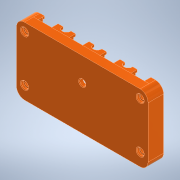
# Autodesk Inventor part: casing-top
Saved by Autodesk Inventor 2021 (Build 250183000, 183)
## iProperties
Created: 2022-04-08
Part Number: casing-top
Material: PET Plastic
Document SubType Name: Modeling
Designer: Staňa
Density: 1.541 g/cm^3
Appearance: Smooth - Light Orange
Author: Staňa
Autodesk Inventor part; units mm, degrees
ref_plane "YZ Plane" through (0, 0, 0) normal (1, 0, 0) x (0, 1, 0)
ref_plane "XZ Plane" through (0, 0, 0) normal (0, 1, 0) x (-1, 0, 0)
ref_plane "XY Plane" through (0, 0, 0) normal (0, 0, 1) x (1, 0, 0)
sketch "Sketch1" plane through (0, 0, 0) normal (0, 0, 1) x (1, 0, 0)
  line L0 (-46.7497, 20.955) -> (-42.9801, 20.955) construction
  line L1 (-42.9801, 20.955) -> (-42.9801, 22.455) construction
  line L2 (-42.9801, 22.455) -> (-46.7497, 22.455) projected
  arc A0 (-46.7497, 22.455) -> (-51.75, 17.4547) centre (-46.7497, 17.4547) ccw projected
  line L3 (-51.75, 17.4547) -> (-51.75, -19.9997) projected
  arc A1 (-51.75, -19.9997) -> (-46.7497, -25) centre (-46.7497, -19.9997) ccw projected
  line L4 (-46.7497, -25) -> (-35.7299, -25) projected
  line L5 (-35.7299, -25) -> (-35.7299, -23.5) construction
  line L6 (-35.7299, -23.5) -> (-46.7497, -23.5) construction
  arc A2 (-50.25, -19.9997) -> (-46.7497, -23.5) centre (-46.7497, -19.9997) ccw construction
  line L7 (-50.25, -19.9997) -> (-50.25, 17.4547) construction
  arc A3 (-46.7497, 20.955) -> (-50.25, 17.4547) centre (-46.7497, 17.4547) ccw construction
  line L8 (-27.98, 20.955) -> (-27.98, 22.455) construction
  line L9 (-27.98, 22.455) -> (-32.0201, 22.455) projected
  line L10 (-32.0201, 22.455) -> (-32.0201, 20.955) construction
  line L11 (-32.0201, 20.955) -> (-27.98, 20.955) construction
  line L12 (-21.63, 22.455) -> (-21.63, 20.955) construction
  line L13 (-21.63, 20.955) -> (-17.9801, 20.955) construction
  line L14 (-17.9801, 20.955) -> (-17.9801, 22.455) construction
  line L15 (-17.9801, 22.455) -> (-21.63, 22.455) projected
  line L16 (-2.98, 20.955) -> (-2.98, 22.455) construction
  line L17 (-2.98, 22.455) -> (-7.0201, 22.455) projected
  line L18 (-7.0201, 22.455) -> (-7.0201, 20.955) construction
  line L19 (-7.0201, 20.955) -> (-2.98, 20.955) construction
  line L20 (3.37, 22.455) -> (3.37, 20.955) construction
  line L21 (3.37, 20.955) -> (7.0199, 20.955) construction
  line L22 (7.0199, 20.955) -> (7.0199, 22.455) construction
  line L23 (7.0199, 22.455) -> (3.37, 22.455) projected
  line L24 (22.02, 20.955) -> (22.02, 22.455) construction
  line L25 (22.02, 22.455) -> (17.9799, 22.455) projected
  line L26 (17.9799, 22.455) -> (17.9799, 20.955) construction
  line L27 (17.9799, 20.955) -> (22.02, 20.955) construction
  line L28 (28.37, 22.455) -> (28.37, 20.955) construction
  line L29 (28.37, 20.955) -> (32.0199, 20.955) construction
  line L30 (32.0199, 20.955) -> (32.0199, 22.455) construction
  line L31 (32.0199, 22.455) -> (28.37, 22.455) projected
  line L32 (50.25, 17.4547) -> (50.25, -19.9997) construction
  arc A4 (46.7497, -23.5) -> (50.25, -19.9997) centre (46.7497, -19.9997) ccw construction
  line L33 (46.7497, -23.5) -> (35.7301, -23.5) construction
  line L34 (35.7301, -23.5) -> (35.7301, -25) construction
  line L35 (35.7301, -25) -> (46.7497, -25) projected
  arc A5 (46.7497, -25) -> (51.75, -19.9997) centre (46.7497, -19.9997) ccw projected
  line L36 (51.75, -19.9997) -> (51.75, 17.4547) projected
  arc A6 (51.75, 17.4547) -> (46.7497, 22.455) centre (46.7497, 17.4547) ccw projected
  line L37 (46.7497, 22.455) -> (42.9799, 22.455) projected
  line L38 (42.9799, 22.455) -> (42.9799, 20.955) construction
  line L39 (42.9799, 20.955) -> (46.7497, 20.955) construction
  arc A7 (50.25, 17.4547) -> (46.7497, 20.955) centre (46.7497, 17.4547) ccw construction
  arc A8 (-46.7497, 24.2499) -> (-53.25, 17.7496) centre (-46.7497, 17.7496) ccw projected
  line L40 (-53.25, 17.7496) -> (-53.25, -23.7996) projected
  arc A9 (-53.25, -23.7996) -> (-46.7497, -30.2999) centre (-46.7497, -23.7996) ccw projected
  line L41 (-46.7497, -30.2999) -> (46.7497, -30.2999) projected
  arc A10 (46.7497, -30.2999) -> (53.25, -23.7996) centre (46.7497, -23.7996) ccw projected
  line L42 (53.25, -23.7996) -> (53.25, 17.7496) projected
  arc A11 (53.25, 17.7496) -> (46.7497, 24.2499) centre (46.7497, 17.7496) ccw projected
  line L43 (46.7497, 24.2499) -> (42.9799, 24.2499)
  line L44 (42.9799, 24.2499) -> (42.9799, 22.455)
  line L45 (-46.7497, 24.2499) -> (-42.9801, 24.2499)
  line L46 (-42.9801, 24.2499) -> (-42.9801, 22.455)
  line L47 (-35.7299, -25) -> (-35.7299, -30.2999)
  line L48 (35.7301, -25) -> (35.7301, -30.2999)
  line L49 (-32.0201, 22.455) -> (-17.9801, 22.455)
  line L50 (-17.9801, 22.455) -> (-17.9801, 24.2499)
  line L51 (-17.9801, 24.2499) -> (-32.0201, 24.2499)
  line L52 (-32.0201, 24.2499) -> (-32.0201, 22.455)
  line L53 (-7.0201, 22.455) -> (7.0199, 22.455)
  line L54 (7.0199, 22.455) -> (7.0199, 24.2499)
  line L55 (7.0199, 24.2499) -> (-7.0201, 24.2499)
  line L56 (-7.0201, 24.2499) -> (-7.0201, 22.455)
  line L57 (17.9799, 22.455) -> (32.0199, 22.455)
  line L58 (32.0199, 22.455) -> (32.0199, 24.2499)
  line L59 (32.0199, 24.2499) -> (17.9799, 24.2499)
  line L60 (17.9799, 24.2499) -> (17.9799, 22.455)
  constraints: 36 end point, 7 perpendicular, 6 parallel, 5 horizontal, 5 point on line, 3 collinear
extrude "bottom-indent" add sketch "Sketch1" along normal blind 1.5
sketch "Sketch3" plane through (0, 0, 1.5) normal (0, 0, 1) x (1, 0, 0)
  arc A0 (-51.75, -19.9997) -> (-46.7497, -25) centre (-46.7497, -19.9997) ccw
  line L0 (-51.75, -19.9997) -> (-51.75, 17.4547)
  arc A1 (-46.7497, 22.455) -> (-51.75, 17.4547) centre (-46.7497, 17.4547) ccw
  line L1 (-46.7497, 22.455) -> (-42.9801, 22.455) construction
  line L2 (-42.9801, 22.455) -> (-42.9801, 24.2499)
  line L3 (-42.9801, 24.2499) -> (-46.7497, 24.2499)
  arc A2 (-46.7497, 24.2499) -> (-53.25, 17.7496) centre (-46.7497, 17.7496) ccw
  line L4 (-53.25, 17.7496) -> (-53.25, -23.7996)
  arc A3 (-53.25, -23.7996) -> (-46.7497, -30.2999) centre (-46.7497, -23.7996) ccw
  line L5 (-46.7497, -30.2999) -> (-35.7299, -30.2999)
  line L6 (-35.7299, -30.2999) -> (-35.7299, -25)
  line L7 (-35.7299, -25) -> (-46.7497, -25)
  line L8 (-46.7497, 20.955) -> (-42.9801, 20.955)
  line L9 (-42.9801, 20.955) -> (-42.9801, 22.455)
  line L10 (-42.9801, 22.455) -> (-46.7497, 22.455) construction
  arc A4 (-46.7497, 22.455) -> (-51.75, 17.4547) centre (-46.7497, 17.4547) ccw
  line L11 (-51.75, 17.4547) -> (-51.75, -19.9997)
  arc A5 (-51.75, -19.9997) -> (-46.7497, -25) centre (-46.7497, -19.9997) ccw
  line L12 (-46.7497, -25) -> (-35.7299, -25)
  line L13 (-35.7299, -25) -> (-35.7299, -23.5)
  line L14 (-35.7299, -23.5) -> (-46.7497, -23.5)
  arc A6 (-50.25, -19.9997) -> (-46.7497, -23.5) centre (-46.7497, -19.9997) ccw
  line L15 (-50.25, -19.9997) -> (-50.25, 17.4547)
  arc A7 (-46.7497, 20.955) -> (-50.25, 17.4547) centre (-46.7497, 17.4547) ccw
  line L16 (-32.0201, 22.455) -> (-17.9801, 22.455) construction
  line L17 (-17.9801, 22.455) -> (-17.9801, 24.2499)
  line L18 (-17.9801, 24.2499) -> (-32.0201, 24.2499)
  line L19 (-32.0201, 24.2499) -> (-32.0201, 22.455)
  line L20 (-7.0201, 22.455) -> (7.0199, 22.455) construction
  line L21 (7.0199, 22.455) -> (7.0199, 24.2499)
  line L22 (7.0199, 24.2499) -> (-7.0201, 24.2499)
  line L23 (-7.0201, 24.2499) -> (-7.0201, 22.455)
  line L24 (17.9799, 22.455) -> (32.0199, 22.455) construction
  line L25 (32.0199, 22.455) -> (32.0199, 24.2499)
  line L26 (32.0199, 24.2499) -> (17.9799, 24.2499)
  line L27 (17.9799, 24.2499) -> (17.9799, 22.455)
  line L28 (35.7301, -25) -> (35.7301, -30.2999)
  line L29 (35.7301, -30.2999) -> (46.7497, -30.2999)
  arc A8 (46.7497, -30.2999) -> (53.25, -23.7996) centre (46.7497, -23.7996) ccw
  line L30 (53.25, -23.7996) -> (53.25, 17.7496)
  arc A9 (53.25, 17.7496) -> (46.7497, 24.2499) centre (46.7497, 17.7496) ccw
  line L31 (46.7497, 24.2499) -> (42.9799, 24.2499)
  line L32 (42.9799, 24.2499) -> (42.9799, 22.455)
  line L33 (42.9799, 22.455) -> (46.7497, 22.455) construction
  arc A10 (51.75, 17.4547) -> (46.7497, 22.455) centre (46.7497, 17.4547) ccw
  line L34 (51.75, 17.4547) -> (51.75, -19.9997)
  arc A11 (46.7497, -25) -> (51.75, -19.9997) centre (46.7497, -19.9997) ccw
  line L35 (46.7497, -25) -> (35.7301, -25)
  line L36 (50.25, 17.4547) -> (50.25, -19.9997)
  arc A12 (46.7497, -23.5) -> (50.25, -19.9997) centre (46.7497, -19.9997) ccw
  line L37 (46.7497, -23.5) -> (35.7301, -23.5)
  line L38 (35.7301, -23.5) -> (35.7301, -25)
  line L39 (35.7301, -25) -> (46.7497, -25)
  arc A13 (46.7497, -25) -> (51.75, -19.9997) centre (46.7497, -19.9997) ccw
  line L40 (51.75, -19.9997) -> (51.75, 17.4547)
  arc A14 (51.75, 17.4547) -> (46.7497, 22.455) centre (46.7497, 17.4547) ccw
  line L41 (46.7497, 22.455) -> (42.9799, 22.455) construction
  line L42 (42.9799, 22.455) -> (42.9799, 20.955)
  line L43 (42.9799, 20.955) -> (46.7497, 20.955)
  arc A15 (50.25, 17.4547) -> (46.7497, 20.955) centre (46.7497, 17.4547) ccw
  line L44 (-32.0201, 24.2499) -> (-32.0201, 22.455)
  line L45 (-32.0201, 24.2499) -> (-17.9801, 24.2499)
  line L46 (-17.9801, 24.2499) -> (-17.9801, 20.955)
  line L47 (-17.9801, 20.955) -> (-32.0201, 20.955)
  line L48 (-32.0201, 20.955) -> (-32.0201, 24.2499)
  line L49 (-17.9801, 22.455) -> (-17.9801, 24.2499)
  line L50 (7.0199, 24.2499) -> (-7.0201, 24.2499)
  line L51 (-7.0201, 24.2499) -> (7.0199, 24.2499)
  line L52 (7.0199, 24.2499) -> (7.0199, 20.955)
  line L53 (7.0199, 20.955) -> (-7.0201, 20.955)
  line L54 (-7.0201, 20.955) -> (-7.0201, 24.2499)
  line L55 (32.0199, 24.2499) -> (17.9799, 24.2499)
  line L56 (17.9799, 24.2499) -> (32.0199, 24.2499)
  line L57 (32.0199, 24.2499) -> (32.0199, 20.955)
  line L58 (32.0199, 20.955) -> (17.9799, 20.955)
  line L59 (17.9799, 20.955) -> (17.9799, 24.2499)
  line L60 (32.0199, 22.455) -> (32.0199, 24.2499)
  line L61 (7.0199, 22.455) -> (7.0199, 24.2499)
  point P0 (0, 0)
extrude "dut-conn-wall" add sketch "Sketch3" along normal blind 3.7
sketch "Sketch4" plane through (0, 0, 5.2) normal (0, 0, 1) x (1, 0, 0)
  line L0 (-35.7299, -23.5) -> (-46.7497, -23.5) projected
  arc A0 (-50.25, -19.9997) -> (-46.7497, -23.5) centre (-46.7497, -19.9997) ccw projected
  line L1 (-50.25, -19.9997) -> (-50.25, 17.4547) projected
  arc A1 (-46.7497, 20.955) -> (-50.25, 17.4547) centre (-46.7497, 17.4547) ccw projected
  line L2 (-46.7497, 20.955) -> (-42.9801, 20.955) projected
  line L3 (-42.9801, 20.955) -> (-42.9801, 24.2499) construction
  line L4 (-42.9801, 24.2499) -> (-46.7497, 24.2499) projected
  arc A2 (-46.7497, 24.2499) -> (-53.25, 17.7496) centre (-46.7497, 17.7496) ccw projected
  line L5 (-53.25, 17.7496) -> (-53.25, -23.7996) projected
  arc A3 (-53.25, -23.7996) -> (-46.7497, -30.2999) centre (-46.7497, -23.7996) ccw projected
  line L6 (-46.7497, -30.2999) -> (-35.7299, -30.2999) projected
  line L7 (-35.7299, -30.2999) -> (-35.7299, -23.5) projected
  line L8 (35.7301, -30.2999) -> (46.7497, -30.2999) projected
  arc A4 (46.7497, -30.2999) -> (53.25, -23.7996) centre (46.7497, -23.7996) ccw projected
  line L9 (53.25, -23.7996) -> (53.25, 17.7496) projected
  arc A5 (53.25, 17.7496) -> (46.7497, 24.2499) centre (46.7497, 17.7496) ccw projected
  line L10 (46.7497, 24.2499) -> (42.9799, 24.2499) projected
  line L11 (42.9799, 24.2499) -> (42.9799, 20.955) construction
  line L12 (42.9799, 20.955) -> (46.7497, 20.955) projected
  arc A6 (50.25, 17.4547) -> (46.7497, 20.955) centre (46.7497, 17.4547) ccw projected
  line L13 (50.25, 17.4547) -> (50.25, -19.9997) projected
  arc A7 (46.7497, -23.5) -> (50.25, -19.9997) centre (46.7497, -19.9997) ccw projected
  line L14 (46.7497, -23.5) -> (35.7301, -23.5) projected
  line L15 (35.7301, -23.5) -> (35.7301, -30.2999) projected
  line L16 (-42.9801, 24.2499) -> (-46.7497, 24.2499) projected
  line L17 (46.7497, 24.2499) -> (42.9799, 24.2499) projected
  line L18 (-42.9801, 24.2499) -> (42.9799, 24.2499)
  line L19 (42.9799, 20.955) -> (-42.9801, 20.955)
  point P0 (0, 0)
  constraints: 4 end point, 1 collinear, 1 horizontal
extrude "mso-conn-wall" add sketch "Sketch4" along normal blind 4.15
sketch "Sketch5" plane through (0, 0, 9.35) normal (0, 0, 1) x (1, 0, 0)
  line L0 (46.7497, 24.2499) -> (-46.7497, 24.2499) projected
  arc A0 (-46.7497, 24.2499) -> (-53.25, 17.7496) centre (-46.7497, 17.7496) ccw projected
  line L1 (-53.25, 17.7496) -> (-53.25, -23.7996) projected
  arc A1 (-53.25, -23.7996) -> (-46.7497, -30.2999) centre (-46.7497, -23.7996) ccw projected
  line L2 (-46.7497, -30.2999) -> (-35.7299, -30.2999) projected
  line L3 (-35.7299, -30.2999) -> (-35.7299, -23.5) construction
  line L4 (-35.7299, -23.5) -> (-46.7497, -23.5) projected
  arc A2 (-50.25, -19.9997) -> (-46.7497, -23.5) centre (-46.7497, -19.9997) ccw projected
  line L5 (-50.25, -19.9997) -> (-50.25, 17.4547) projected
  arc A3 (-46.7497, 20.955) -> (-50.25, 17.4547) centre (-46.7497, 17.4547) ccw projected
  line L6 (-46.7497, 20.955) -> (46.7497, 20.955) projected
  arc A4 (50.25, 17.4547) -> (46.7497, 20.955) centre (46.7497, 17.4547) ccw projected
  line L7 (50.25, 17.4547) -> (50.25, -19.9997) projected
  arc A5 (46.7497, -23.5) -> (50.25, -19.9997) centre (46.7497, -19.9997) ccw projected
  line L8 (46.7497, -23.5) -> (35.7301, -23.5) projected
  line L9 (35.7301, -23.5) -> (35.7301, -30.2999) construction
  line L10 (35.7301, -30.2999) -> (46.7497, -30.2999) projected
  arc A6 (46.7497, -30.2999) -> (53.25, -23.7996) centre (46.7497, -23.7996) ccw projected
  line L11 (53.25, -23.7996) -> (53.25, 17.7496) projected
  arc A7 (53.25, 17.7496) -> (46.7497, 24.2499) centre (46.7497, 17.7496) ccw projected
  line L12 (-46.7497, -30.2999) -> (-35.7299, -30.2999) projected
  line L13 (-35.7299, -30.2999) -> (35.7301, -30.2999)
  line L14 (-35.7299, -23.5) -> (-46.7497, -23.5) construction
  line L15 (-35.7299, -30.2999) -> (-35.7299, -23.5) construction
  line L16 (-35.7299, -23.5) -> (-46.7497, -23.5) projected
  line L17 (46.7497, -23.5) -> (35.7301, -23.5) projected
  point P0 (0, 0)
  constraints: 2 end point, 1 horizontal
extrude "roof" add sketch "Sketch5" along normal blind 3.15
sketch "Sketch7" plane through (-7.0201, 24.2499, 0) normal (0, 1, 0) x (1, 0, 0)
  circle A0 centre (32.0201, -0.255) radius 3.25 construction
  arc A1 (29.2901, -1.7655) -> (29.2901, 1.2555) centre (32.0201, -0.255) ccw construction
  line L0 (29.2901, -1.7655) -> (29.2901, 1.2555) construction
  circle A2 centre (7.0201, -0.255) radius 3.25 construction
  arc A3 (4.2901, -1.7655) -> (4.2901, 1.2555) centre (7.0201, -0.255) ccw construction
  line L1 (4.2901, -1.7655) -> (4.2901, 1.2555) construction
  circle A4 centre (-17.9799, -0.255) radius 3.25 construction
  arc A5 (-20.7099, -1.7655) -> (-20.7099, 1.2555) centre (-17.9799, -0.255) ccw construction
  line L2 (-20.7099, -1.7655) -> (-20.7099, 1.2555) construction
  arc A6 (29.0401, -1.8287) -> (29.0401, 1.3187) centre (32.0201, -0.255) ccw
  line L3 (29.0401, -1.8287) -> (29.0401, 1.3187)
  arc A7 (4.0401, -1.8287) -> (4.0401, 1.3187) centre (7.0201, -0.255) ccw
  line L4 (4.0401, -1.8287) -> (4.0401, 1.3187)
  arc A8 (-20.9599, -1.8287) -> (-20.9599, 1.3187) centre (-17.9799, -0.255) ccw
  line L5 (-20.9599, -1.8287) -> (-20.9599, 1.3187)
  point P0 (7.0201, 0)
  dimension "d17" = 0.25
  dimension "d18" = 0.25
  dimension "d19" = 0.25
  constraints: 6 end point, 6 point on circle, 3 centre point, 3 other
  measures "d17" distance between parallel lines of L0 L3
  measures "d18" radial gap between concentric circles of A3 A7
  measures "d19" radial gap between concentric circles of A5 A8
extrude "coax-cutout" cut sketch "Sketch7" against normal up to surface (3.2949 mm away)
sketch "Sketch8" plane through (0, 0, 9.35) normal (0, 0, -1) x (-1, 0, 0)
  line L0 (-35.7301, -23.5) -> (-35.7301, -30.2999) projected
  line L1 (35.7299, -30.2999) -> (-35.7301, -30.2999) projected
  line L2 (35.7299, -30.2999) -> (35.7299, -23.5) projected
  line L3 (35.7299, -23.5) -> (46.7497, -23.5) projected
  arc A0 (46.7497, -23.5) -> (50.25, -19.9997) centre (46.7497, -19.9997) ccw projected
  line L4 (50.25, -19.9997) -> (50.25, 17.4547) projected
  arc A1 (50.25, 17.4547) -> (46.7497, 20.955) centre (46.7497, 17.4547) ccw projected
  line L5 (46.7497, 20.955) -> (-46.7497, 20.955) projected
  arc A2 (-46.7497, 20.955) -> (-50.25, 17.4547) centre (-46.7497, 17.4547) ccw projected
  line L6 (-50.25, 17.4547) -> (-50.25, -19.9997) projected
  arc A3 (-50.25, -19.9997) -> (-46.7497, -23.5) centre (-46.7497, -19.9997) ccw projected
  line L7 (-46.7497, -23.5) -> (-35.7301, -23.5) projected
  line L8 (0, 41.7757) -> (0, -44.7611) construction
  arc A4 (43.2493, 17.4547) -> (46.7497, 13.9543) centre (46.7497, 17.4547) ccw
  circle A5 centre (46.75, 17.455) radius 1.6 construction
  circle A6 centre (46.75, -20) radius 1.6 construction
  line L9 (46.7497, 13.9543) -> (48.35, 13.9543)
  line L10 (48.35, 13.9543) -> (48.35, 17.455) construction
  line L11 (43.2493, 17.4547) -> (43.2493, 19.055)
  line L12 (43.2493, 19.055) -> (46.75, 19.055) construction
  arc A7 (46.75, -16.4997) -> (43.2497, -20) centre (46.75, -20) ccw
  line L13 (43.2497, -20) -> (43.2497, -21.6)
  line L14 (43.2497, -21.6) -> (46.75, -21.6) construction
  line L15 (46.75, -16.4997) -> (48.35, -16.4997)
  line L16 (48.35, -16.4997) -> (48.35, -20) construction
  line L17 (42.9801, 20.955) -> (32.0201, 20.955) projected
  arc A8 (43.2493, 19.055) -> (41.3493, 20.955) centre (41.3493, 19.055) ccw
  line L18 (50.25, -19.9997) -> (50.25, 17.4547) projected
  arc A9 (50.25, 12.0543) -> (48.35, 13.9543) centre (48.35, 12.0543) ccw
  arc A10 (48.35, -16.4997) -> (50.25, -14.5997) centre (48.35, -14.5997) ccw
  line L19 (35.7299, -23.5) -> (46.7497, -23.5) projected
  arc A11 (41.3497, -23.5) -> (43.2497, -21.6) centre (41.3497, -21.6) ccw
  arc A12 (-46.7497, 13.9543) -> (-43.2493, 17.4547) centre (-46.7497, 17.4547) ccw
  line L20 (-46.7497, 13.9543) -> (-48.35, 13.9543)
  line L21 (-43.2493, 17.4547) -> (-43.2493, 19.055)
  arc A13 (-43.2497, -20) -> (-46.75, -16.4997) centre (-46.75, -20) ccw
  line L22 (-43.2497, -20) -> (-43.2497, -21.6)
  line L23 (-46.75, -16.4997) -> (-48.35, -16.4997)
  arc A14 (-41.3493, 20.955) -> (-43.2493, 19.055) centre (-41.3493, 19.055) ccw
  arc A15 (-48.35, 13.9543) -> (-50.25, 12.0543) centre (-48.35, 12.0543) ccw
  arc A16 (-50.25, -14.5997) -> (-48.35, -16.4997) centre (-48.35, -14.5997) ccw
  arc A17 (-43.2497, -21.6) -> (-41.3497, -23.5) centre (-41.3497, -21.6) ccw
  point P0 (0, 0)
  point P1 (-41.3497, -23.5)
  point P2 (-50.25, -14.5997)
  point P3 (-50.25, 12.0543)
  point P4 (-41.3493, 20.955)
  point P5 (41.3493, 20.955)
  point P6 (50.25, 12.0544)
  point P7 (50.25, -14.5997)
  point P8 (41.3497, -23.5)
  dimension "d31" = 3.5003
  constraints: 28 point on circle, 26 end point, 18 symmetric about line, 16 tangent, 12 centre point, 5 point on line, 4 perpendicular, 3 vertical, 2 coincident, 2 horizontal, 1 equal radius, 6 other
  measures "d31" radius of A4
extrude "spacer-support" add sketch "Sketch8" along normal blind 1.35 contours L7 A3 L6 A16 L23 A13 L22 A17 | A11 L13 A7 L15 A10 L4 A0 L3 | L6 A2 L5 A14 L21 A12 L20 A15 | A9 L9 A4 L11 A8 L5 A1 L4
fillet "spacer-support-fillet" radius 0.5 24 edges at (-49.6935, 13.3979, 9.35) (-47.5498, 13.9543, 9.35) (-44.2746, 14.9796, 9.35) (-43.2493, 18.2548, 9.35) (-42.6928, 20.3985, 9.35) (42.6928, 20.3985, 9.35) (43.2493, 18.2548, 9.35) (44.2746, 14.9796, 9.35) (47.5498, 13.9543, 9.35) (49.6935, 13.3978, 9.35) (50.25, -1.2727, 9.35) (49.6935, -15.9432, 9.35) (47.55, -16.4997, 9.35) (44.2749, -17.5249, 9.35) (43.2497, -20.8, 9.35) (42.6932, -22.9435, 9.35) (38.5399, -23.5, 9.35) (-49.6935, -15.9432, 9.35) (-47.55, -16.4997, 9.35) (-44.2749, -17.5249, 9.35) (-43.2497, -20.8, 9.35) (-42.6932, -22.9435, 9.35) (-38.5398, -23.5, 9.35) (-50.25, -1.2727, 9.35)
sketch "Sketch9" plane through (0, 0, 12.5) normal (0, 0, 1) x (1, 0, 0)
  circle A0 centre (-46.75, -20) radius 1.6 construction
  circle A1 centre (-46.75, 17.455) radius 1.6 construction
  circle A2 centre (46.75, 17.455) radius 1.6 construction
  circle A3 centre (46.75, -20) radius 1.6 construction
hole "screw-holes" at (-46.75, 17.455, 12.5) at (-46.75, -20, 12.5) at (46.75, 17.455, 12.5) at (46.75, -20, 12.5) direction (0, 0, -1) diameter 3.4 end through all counterbore diameter 5.7 counterbore depth 2 clearance for "Hex Head Cap Screw ISO 24017" size "M3" standard "ISO"
sketch "Sketch10" plane through (0, 0, 12.5) normal (0, 0, 1) x (1, 0, 0)
  circle A0 centre (-0.0001, 5) radius 2.5 projected
  point P0 (0, 0)
extrude "led-hole" cut sketch "Sketch10" against normal through all
chamfer "top-hole-chamfer" distance 0.5 angle 45 5 edges at (-2.5001, 5, 12.5) (-46.75, -17.15, 12.5) (46.75, -17.15, 12.5) (-46.75, 20.305, 12.5) (46.75, 20.305, 12.5)
equation "\"d18\" = d17"
equation "\"d19\" = d17"
body "Solid1"
